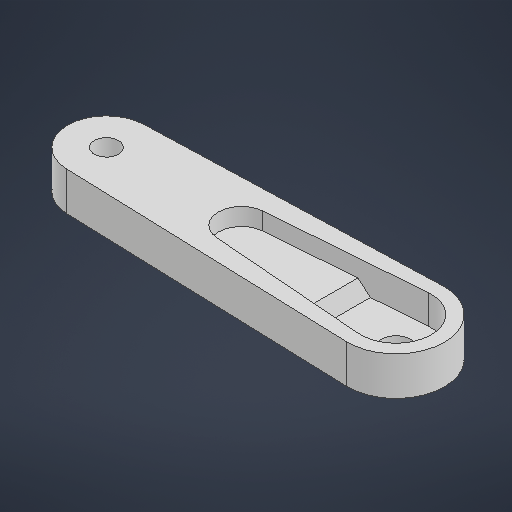
# Autodesk Inventor part: Servo Arm
Saved by Autodesk Inventor 2025.1 (Build 291241000, 241)
## iProperties
Created: 2025-03-13
Part Number: Servo Arm
Material: Generic
Document SubType Name: Modeling
Designer: jerem
Density: 1 g/cm^3
Appearance: Default
Author: jerem
## iProperties of the stored document Servo Arm_3DPrint.ipt
Created: 2025-03-13
Part Number: Servo Arm_3DPrint
Material: Generic
Document SubType Name: Modeling
Designer: jerem
Density: 1 g/cm^3
Appearance: Default
Author: jerem
Autodesk Inventor part; units mm, degrees
ref_plane "YZ Plane" through (0, 0, 0) normal (1, 0, 0) x (0, 1, 0)
ref_plane "XZ Plane" through (0, 0, 0) normal (0, 1, 0) x (-1, 0, 0)
ref_plane "XY Plane" through (0, 0, 0) normal (0, 0, 1) x (1, 0, 0)
sketch "Sketch1" plane through (0, 0, 0) normal (0, 1, 0) x (-1, 0, 0)
  arc A0 (0.2852, 3.6388) -> (0.2852, -3.6388) centre (0, 0) ccw
  line L0 (0, 0) -> (16, 0) construction
  arc A1 (16.1875, -2.3927) -> (16.1875, 2.3927) centre (16, 0) ccw
  line L1 (0.2852, 3.6388) -> (16.1875, 2.3927)
  line L2 (0.2852, -3.6388) -> (16.1875, -2.3927)
  line L3 (5.85, 3.2028) -> (5.85, -3.2028)
  line L4 (0, 0) -> (-3.65, 0)
  circle A2 centre (0, 0) radius 1.55
  circle A3 centre (0, 0) radius 3
  circle A4 centre (0, 0) radius 5
  line L5 (0.1667, 4.9972) -> (30.1333, 3.9978)
  line L6 (0.1667, -4.9972) -> (30.1333, -3.9978)
  circle A5 centre (30, 0) radius 4
  line L7 (16, 0) -> (30, 0) construction
  circle A6 centre (30, 0) radius 1.25
  point P0 (0, 0)
  dimension "d0" = 7.3
  dimension "d1" = 4.8
  dimension "d2" = 16
  dimension "d3" = 9.5
  dimension "d4" = 3.1
  dimension "d6" = 6
  dimension "d8" = 2.5
  dimension "d18" = 10
  dimension "d19" = 8
  dimension "d20" = 30
  constraints: 17 end point, 9 point on circle, 8 tangent, 7 centre point, 7 coincident, 3 horizontal, 2 point on line, 1 vertical
  measures "d0" diameter of A0
  measures "d1" diameter of A1
  measures "d2" distance of L0.end point (0, 0)
  measures "d3" distance from line of L4.end L3
  measures "d4" diameter of A2
  measures "d6" diameter of A3
  measures "d8" diameter of A6
  measures "d18" diameter of A4
  measures "d19" diameter of A5
  measures "d20" distance of L7.end point (0, 0)
extrude "Extrusion1" add sketch "Sketch1" against normal blind 1 contours A3 | L1 A4 L2 A0 | A0 L2 A4 L1 | A4 L5 A5 L6 L2 A1 L1 | L1 L3 L2 A4 | L1 A1 L2 L3 | A5
extrude "Extrusion2" add sketch "Sketch1" along normal blind 3 contours A0 L2 A4 L1 | A4 L5 A5 L6 L2 A1 L1 | A5 picked at (2.3095, 3.6823)
extrude "Extrusion3" add sketch "Sketch1" along normal blind 1.2 contours L1 A1 L2 L3
chamfer "Chamfer1" distance 1.2 angle 45 1 edges at (-5.85, 1.2, 0)
body "Solid1"
